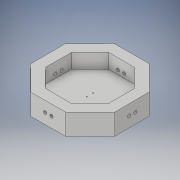
# Autodesk Inventor part: oktagonOben
Saved by Autodesk Inventor 2019 (Build 230136000, 136)
## iProperties
Created: 2018-08-07
Part Number: oktagonOben
Material: Generic
Document SubType Name: Modeling
Designer: chris
Density: 1 g/cm^3
Appearance: Default
Author: chris
Autodesk Inventor part; units mm, degrees
ref_plane "YZ Plane" through (0, 0, 0) normal (1, 0, 0) x (0, 1, 0)
ref_plane "XZ Plane" through (0, 0, 0) normal (0, 1, 0) x (-1, 0, 0)
ref_plane "XY Plane" through (0, 0, 0) normal (0, 0, 1) x (1, 0, 0)
sketch "Sketch2" plane through (0, 0, 0) normal (0, 1, 0) x (-1, 0, 0)
  line L0 (8.4085, -19.9481) -> (-8.1597, -20.0511)
  line L1 (-8.1597, -20.0511) -> (-19.9481, -8.4085)
  line L2 (-19.9481, -8.4085) -> (-20.0511, 8.1597)
  line L3 (-20.0511, 8.1597) -> (-8.4085, 19.9481)
  line L4 (-8.4085, 19.9481) -> (8.1597, 20.0511)
  line L5 (8.1597, 20.0511) -> (19.9481, 8.4085)
  line L6 (19.9481, 8.4085) -> (20.0511, -8.1597)
  line L7 (20.0511, -8.1597) -> (8.4085, -19.9481)
  point P0 (0, 0)
  point P1 (0, 0)
  dimension "d12" = 20
  dimension "d13" = 16.5682
  constraints: 16 end point, 1 coincident, 17 other
  measures "d12" distance from line of L0 point (0, 0)
  measures "d13" horizontal distance of L3.end L4.end
extrude "Extrusion1" add sketch "Sketch2" along normal blind 10
sketch "Sketch3" plane through (0, 10, 0) normal (0, 1, 0) x (1, 0, 0)
  line L0 (-6.1212, 15.0378) -> (6.305, 14.9616)
  line L1 (6.305, 14.9616) -> (15.0378, 6.1212)
  line L2 (15.0378, 6.1212) -> (14.9616, -6.305)
  line L3 (14.9616, -6.305) -> (6.1212, -15.0378)
  line L4 (6.1212, -15.0378) -> (-6.305, -14.9616)
  line L5 (-6.305, -14.9616) -> (-15.0378, -6.1212)
  line L6 (-15.0378, -6.1212) -> (-14.9616, 6.305)
  line L7 (-14.9616, 6.305) -> (-6.1212, 15.0378)
  point P0 (0, 0)
  point P1 (0, 0)
  dimension "d16" = 15
  dimension "d17" = 12.4262
  constraints: 16 end point, 1 coincident, 17 other
  measures "d16" distance from line of L0 point (0, 0)
  measures "d17" horizontal distance of L3.end L4.end
extrude "Extrusion2" cut sketch "Sketch3" against normal blind 7
sketch "Sketch4" plane through (0, 0, 0) normal (0, -1, 0) x (1, 0, 0)
  point P0 (0, 0)
  point P1 (0, 1.5)
  point P2 (0, -1.5)
hole "Hole1" at (0, 0, 1.5) at (0, 0, -1.5) direction (0, 1, 0) diameter 0.5 end through all
sketch "Sketch5" plane through (8.4085, 0, 19.9481) normal (0.0062188, 0, 0.9999807) x (0.9999807, 0, -0.0062188)
  line L0 (-8.2843, 0) -> (-8.2843, 10)
  line L1 (-2.2567, 10) -> (-14.6822, 10) projected
  line L2 (0, 0) -> (0, 10) projected
  line L3 (0, 5) -> (-16.5685, 5)
  line L4 (-16.5685, 0) -> (-16.5685, 10) projected
  point P0 (-9.784, 5)
  point P1 (-6.784, 5)
  constraints: 4 end point, 3 point on line, 2 midpoint, 1 vertical
hole "Hole2" at (-1.3753, 5, 20.0089) at (1.6246, 5, 19.9903) direction (-0.0062188, 0, -0.9999807) diameter 1.5 end through all
sketch "Sketch6" plane through (-19.9481, 0, 8.4085) normal (-0.9999807, 0, 0.0062188) x (0.0062188, 0, 0.9999807)
  line L0 (-8.2843, 0) -> (-8.2843, 10)
  line L1 (-2.2567, 10) -> (-14.6822, 10) projected
  line L2 (-16.5685, 0) -> (-16.5685, 10) projected
  line L3 (-16.5685, 5) -> (0, 5)
  line L4 (0, 0) -> (0, 10) projected
  point P0 (-6.784, 5)
  point P1 (-9.784, 5)
  constraints: 4 end point, 3 point on line, 2 midpoint, 1 vertical
hole "Hole3" at (-19.9903, 5, 1.6246) at (-20.0089, 5, -1.3753) direction (0.9999807, 0, -0.0062188) diameter 1.5 end through all
body "Solid1"
